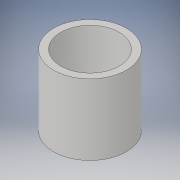
# Autodesk Inventor part: LargeFinderEyePieceCover
Saved by Autodesk Inventor 2019.1 (Build 231200000, 200)
## iProperties
Created: 2018-09-02
Part Number: LargeFinderEyePieceCover
Material: Generic
Document SubType Name: Modeling
Designer: steele
Density: 1 g/cm^3
Appearance: Default
Author: steele
Autodesk Inventor part; units mm, degrees
ref_plane "YZ Plane" through (0, 0, 0) normal (1, 0, 0) x (0, 1, 0)
ref_plane "XZ Plane" through (0, 0, 0) normal (0, 1, 0) x (-1, 0, 0)
ref_plane "XY Plane" through (0, 0, 0) normal (0, 0, 1) x (1, 0, 0)
sketch "Sketch1" plane through (0, 0, 0) normal (0, 1, 0) x (-1, 0, 0)
  circle A0 centre (0, 0) radius 16.337
  dimension "d0" = 32.674
  constraints: 1 centre point, 1 coincident
  measures "d0" diameter of A0
extrude "Extrusion1" add sketch "Sketch1" along normal blind 6.35
sketch "Sketch2" plane through (0, 6.35, 0) normal (0, 1, 0) x (1, 0, 0)
  circle A0 centre (0, 0) radius 16.337
  circle A1 centre (0, 0) radius 13.162
  dimension "d3" = 32.674
  dimension "d4" = 26.324
  constraints: 2 centre point, 2 coincident
  measures "d3" diameter of A0
  measures "d4" diameter of A1
extrude "Extrusion2" add sketch "Sketch2" along normal blind 25.4
equation "\"d0\" = coverOD"
equation "\"d1\" = wallThickness"
equation "\"d3\" = coverOD"
equation "\"d4\" = eypPieceCoverID"
equation "\"wallThickness\" = 6.35"
equation "\"coverOD\" = eypPieceCoverID + wallThickness"
equation "\"eypPieceCoverID\" = 26.324"
body "Solid1"
